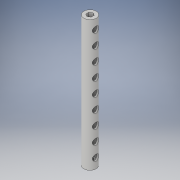
# Autodesk Inventor part: Spinner4inx12mmHex edited 1
Saved by Autodesk Inventor 2019 (Build 230136000, 136)
## iProperties
Created: 2018-09-29
Part Number: Spinner4inx12mmHex edited 1
Material: Generic
Document SubType Name: Modeling
Designer: mrhftc
Density: 1 g/cm^3
Appearance: Default
Author: mrhftc
Autodesk Inventor part; units mm, degrees
ref_plane "YZ Plane" through (0, 0, 0) normal (1, 0, 0) x (0, 1, 0)
sketch "Sketch3" plane through (0, 0, 0) normal (0, 1, 0) x (-1, 0, 0)
  circle A0 centre (0, 0) radius 6
  line L0 (0, 7.3639) -> (0, 0)
  line L1 (0, 0) -> (0, -8.8137)
  line L2 (6.485, 0) -> (0, 0)
  line L3 (-6.963, 0) -> (0, 0)
  line L4 (0, 3.0022) -> (2.6, 1.5011)
  line L5 (0, 3.0022) -> (3.0022, 3.0022) construction
  circle A1 centre (0, 0) radius 6
  line L6 (0, 3.0022) -> (-2.6, 1.5011)
  line L7 (0, -3.0022) -> (2.6, -1.5011)
  line L8 (0, -3.0022) -> (-2.6, -1.5011)
  line L9 (2.6, 1.5011) -> (2.6, -1.5011)
  line L10 (-2.6, 1.5011) -> (-2.6, -1.5011)
  dimension "d6" = 30
  dimension "d7" = 5.2
  dimension "d8" = 3.0022
  dimension "d9" = 3.0022
  dimension "d34" = 12
  constraints: 22 end point, 4 symmetric about line, 3 point on line, 2 centre point, 2 horizontal, 2 vertical, 1 coincident, 1 collinear, 1 equal length, 1 parallel, 1 other
  measures "d6" angle of L4 L5
  measures "d7" distance between parallel lines of L6 L7
  measures "d8" distance of L4.start L4.end
  measures "d9" distance of L4.end L7.end
  measures "d34" diameter of A0
extrude "Extrusion2" add sketch "Sketch3" along normal blind 127 contours L2 L9 L4 L0 A0 | A0 L1 L7 L9 L2 | L0 L6 L10 L3 A0 | A0 L3 L10 L8 L1
ref_plane "Work Plane2" through (6, 0, 0) normal (-1, 0, 0) x (0, -1, 0)
sketch "Sketch4" plane through (6, 0, 0) normal (-1, 0, 0) x (0, -1, 0)
  line L0 (-127, 0) -> (0, 0)
  line L1 (0, 3.0022) -> (-127, 3.0022) projected
  circle A0 centre (-63.5, 0) radius 3
  circle A1 centre (-50, 0) radius 3
  circle A2 centre (-36.5, 0) radius 3
  circle A3 centre (-23, 0) radius 3
  circle A4 centre (-77, 0) radius 3
  circle A5 centre (-63.5, 0) radius 3
  circle A6 centre (-50, 0) radius 3
  circle A7 centre (-36.5, 0) radius 3
  circle A8 centre (-90.5, 0) radius 3
  circle A9 centre (-77, 0) radius 3
  circle A10 centre (-63.5, 0) radius 3
  circle A11 centre (-50, 0) radius 3
  circle A12 centre (-104, 0) radius 3
  circle A13 centre (-90.5, 0) radius 3
  circle A14 centre (-77, 0) radius 3
  circle A15 centre (-63.5, 0) radius 3
  line L2 (-127, 6) -> (-127, -6) construction
  line L3 (-63.5, 42.2406) -> (-63.5, -97.1888) construction
  line L4 (0, -6) -> (0, 6) construction
  circle A16 centre (-9.5, 0) radius 3
  circle A17 centre (-23, 0) radius 3
  circle A18 centre (-36.5, 0) radius 3
  circle A19 centre (-50, 0) radius 3
  circle A20 centre (-117.5, 0) radius 3
  circle A21 centre (-104, 0) radius 3
  circle A22 centre (-90.5, 0) radius 3
  circle A23 centre (-77, 0) radius 3
  circle A24 centre (-63.5, 0) radius 3
  dimension "d17" = 6
  dimension "d20" = 13.5
  dimension "d23" = 13.5
  dimension "d41" = 127
  dimension "d42" = 63.5
  dimension "d43" = 63.5
  constraints: 25 centre point, 4 end point, 2 horizontal, 2 midpoint, 1 parallel, 1 point on line, 1 vertical, 48 other
  measures "d17" diameter of A0
  measures "d20" distance of A0.centre A1.centre
  measures "d23" distance of A0.centre A4.centre
  measures "d41" distance between parallel lines of L4 L2
  measures "d42" distance between parallel lines of L2 L3
  measures "d43" distance between parallel lines of L4 L3
extrude "Main Tube Extrusion" cut sketch "Sketch4" along normal through all
fillet "Inner hex fillets" radius 1 2 edges at (2.6, 26, 0) (-2.6, 26, 0)
ref_plane "Work Plane3" through (0, 5, 0) normal (0, -1, 0) x (1, 0, 0)
sketch "Sketch7" plane through (0, 5, 0) normal (0, -1, 0) x (1, 0, 0)
  circle A0 centre (0, 0) radius 4.5
  dimension "d47" = 9
  constraints: 1 centre point, 1 coincident
  measures "d47" diameter of A0
extrude "Extrusion6" cut sketch "Sketch7" against normal blind 117
equation "\"d8\" = d9"
equation "\"d42\" = 0.5 * d41"
body "Solid2"
